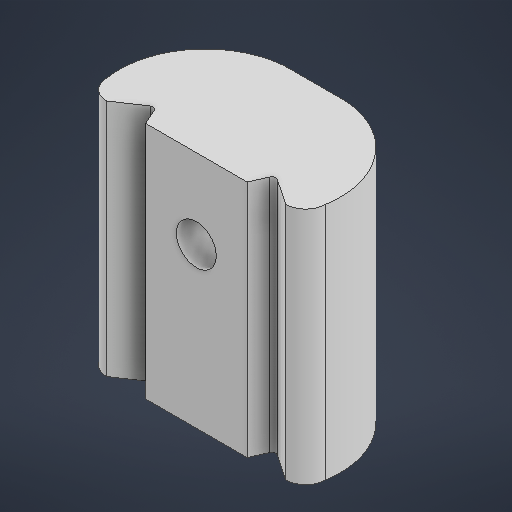
# Autodesk Inventor part: Curved Slider v1.0
Saved by Autodesk Inventor 2027 (Build 310192060, 192F)
## iProperties
Created: 2026-05-20
Part Number: Curved Slider v1.0
Material: Generic
Document SubType Name: Modeling
Designer: cheap
Density: 1 g/cm^3
Appearance: Default
Author: cheap
Autodesk Inventor part; units mm, degrees
ref_plane "YZ Plane" through (0, 0, 0) normal (1, 0, 0) x (0, 1, 0)
ref_plane "XZ Plane" through (0, 0, 0) normal (0, 1, 0) x (-1, 0, 0)
ref_plane "XY Plane" through (0, 0, 0) normal (0, 0, 1) x (1, 0, 0)
sketch "Sketch1" plane through (0, 0, 0) normal (0, 1, 0) x (-1, 0, 0)
  line L0 (2.3057, -4.7625) -> (-8.7313, -4.7625)
  line L1 (-7.1437, 4.7625) -> (7.1438, 4.7625)
  line L2 (8.7313, -4.7625) -> (-8.7313, 4.7625) construction
  line L3 (-8.7313, -4.7625) -> (8.7313, 4.7625) construction
  arc A0 (8.7313, 3.175) -> (7.1438, 4.7625) centre (7.1438, 3.175) ccw
  arc A1 (-7.1437, 4.7625) -> (-8.7313, 3.175) centre (-7.1437, 3.175) ccw
  line L4 (0, -4.7625) -> (-1.5875, -4.7625)
  line L5 (0, -4.7625) -> (1.5875, -4.7625)
  arc A2 (1.5875, -4.7625) -> (8.7313, 3.175) centre (1.9466, 2.0978) ccw
  line L6 (0, -11.8883) -> (0, 12.0323) construction
  arc A3 (-8.7313, 3.175) -> (-1.5875, -4.7625) centre (-1.9466, 2.0978) ccw
  point P0 (0, 0)
  point P1 (-2.3057, -4.7625)
  dimension "d0" = 17.4625
  dimension "d1" = 9.525
  dimension "d2" = 1.5875
  dimension "d3" = 1.5875
  dimension "d4" = 1.5875
  dimension "d5" = 1.5875
  constraints: 14 end point, 9 point on circle, 5 point on line, 4 centre point, 2 midpoint, 2 tangent, 1 horizontal, 1 parallel, 1 symmetric about line, 1 vertical, 1 other
  measures "d0" distance of L2.end L3.end
  measures "d1" distance of L0.end L2.end
  measures "d2" radius of A0
  measures "d3" radius of A1
  measures "d4" distance of L4.start L4.end
  measures "d5" distance of L4.start L5.end
extrude "Extrusion1" add sketch "Sketch1" along normal blind 19.05 contours L0 A3 A1 L1 A0 A2
sketch "Sketch2" plane through (0, 19.05, 0) normal (0, 1, 0) x (1, 0, 0)
  line L0 (-7.1438, -4.7625) -> (7.1437, -4.7625) projected
  line L1 (8.8162, 2.8402) -> (8.8162, -4.7625) construction
  arc A0 (8.7313, -3.175) -> (2.3057, 4.7625) centre (1.9466, -2.0978) ccw construction
  line L2 (4.0537, -4.7625) -> (4.6092, -3.5183)
  line L3 (5.0753, -3.3835) -> (7.1437, -4.7625)
  line L4 (4.0537, -4.7625) -> (7.1437, -4.7625)
  arc A1 (5.0753, -3.3835) -> (4.6092, -3.5183) centre (4.8992, -3.6477) ccw
  line L5 (4.0537, -4.7625) -> (7.1437, -4.7625)
  line L6 (4.0537, -4.7625) -> (7.1437, -4.7625)
  line L7 (2.3057, 4.7625) -> (-2.3057, 4.7625) construction
  line L8 (0, 4.7625) -> (0, -4.7625) construction
  line L9 (-4.0537, -4.7625) -> (-4.6092, -3.5183)
  line L10 (-5.0753, -3.3835) -> (-7.1438, -4.7625)
  line L11 (-4.0537, -4.7625) -> (-7.1438, -4.7625)
  arc A2 (-4.6092, -3.5183) -> (-5.0753, -3.3835) centre (-4.8992, -3.6477) ccw
  line L12 (-4.0537, -4.7625) -> (-7.1438, -4.7625)
  line L13 (-4.0537, -4.7625) -> (-7.1438, -4.7625)
  point P0 (0, 0)
  dimension "d8" = 4.7625
  dimension "d9" = 0.3175
  constraints: 24 end point, 4 point on circle, 4 symmetric about line, 3 tangent, 2 centre point, 2 collinear, 2 midpoint, 1 point on line, 1 vertical, 1 other
  measures "d8" distance from line of L2.start L1
  measures "d9" radius of A1
extrude "Extrusion2" cut sketch "Sketch2" against normal blind 19.05
sketch "Sketch3" plane through (-4.0537, 0, 4.7625) normal (0, 0, 1) x (1, 0, 0)
  circle A0 centre (4.0537, 12.7) radius 1.5875
  line L0 (0, 0) -> (8.1075, 0) projected
  point P0 (4.0537, 0)
  dimension "d12" = 3.175
  dimension "d13" = 12.7
  constraints: 1 centre point
  measures "d12" diameter of A0
  measures "d13" distance from line of L0 A0.centre
extrude "Extrusion3" cut sketch "Sketch3" against normal blind 19.05
body "Solid1"
